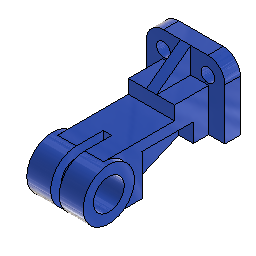
Design 12 v1 (Autodesk Fusion 360 design; units mm, degrees)
Autodesk Fusion 360 part; units mm, degrees
sketch "Sketch1" plane through (0, 0, 0) normal (1, 0, 0) x (0, 1, 0)
  circle A0 centre (0, 0) radius 180
  circle A1 centre (0, 0) radius 300
  line L0 (0, 300) -> (830, 300)
  line L1 (830, 300) -> (830, 460)
  line L2 (830, 460) -> (1230, 460)
  line L3 (1230, 460) -> (1230, -40)
  line L4 (1230, -40) -> (1050, -40)
  line L5 (1050, 180) -> (450, 180)
  line L6 (450, 180) -> (450, -300)
  line L7 (450, -300) -> (0, -300)
  line L8 (1050, 180) -> (1050, -40)
  line L9 (1230, -40) -> (1410, -40)
  line L10 (1410, -40) -> (1410, 760)
  line L11 (1410, 760) -> (1230, 760)
  line L12 (1230, 760) -> (1230, -40)
  line L13 (1230, 760) -> (830, 460)
  line L14 (450, -300) -> (1050, -40)
  dimension "d1" = 360
  dimension "d2" = 600
  dimension "d3" = 800
  dimension "d4" = 180
  dimension "d5" = 180
  dimension "d6" = 450
  dimension "d7" = 600
  dimension "d8" = 160
  dimension "d9" = 120
  dimension "d10" = 220
  dimension "d11" = 400
  dimension "d12" = 480
  constraint coincident A0.centre A1.centre
  constraint concentric A0 A1
  constraint coincident A1 L0.start
  constraint tangent A1 L0
  constraint horizontal L0
  constraint perpendicular L0 L1
  constraint perpendicular L1 L2
  constraint perpendicular L0 L3
  constraint perpendicular L1 L4
  constraint perpendicular L1 L5
  constraint perpendicular L5 L6
  constraint coincident A1 L7.end
  constraint tangent A1 L7
  constraint perpendicular L4 L8
  constraint horizontal L9
  constraint vertical L10
  constraint horizontal L11
  constraint vertical L12
  measures "d1" diameter of A0
  measures "d2" diameter of A1
  measures "d3" distance of L9.end L10.end
  measures "d4" distance of L3.end L9.end
  measures "d5" distance of L3.end L4.end
  measures "d6" horizontal distance of L6.end L7.end
  measures "d7" distance of L5.start L5.end
  measures "d8" distance of L0.end L1.end
  measures "d9" distance of L0 L5
  measures "d10" distance of L4.end L5.start
  measures "d11" distance of L1.end L2.end
  measures "d12" distance of L5.end L6.end
extrude "Extrude1" add sketch "Sketch1" along normal mid plane 660 contours A1
extrude "Extrude2" add sketch "Sketch1" along normal mid plane 540 contours A1 L0 L1 L2 L3 L4 L5 L6 L7 L8 L12
extrude "Extrude3" add sketch "Sketch1" along normal mid plane 120 contours L2 L12 L13
extrude "Extrude4" add sketch "Sketch1" along normal mid plane 920 contours L3 L9 L10 L11 L12
extrude "Extrude5" add sketch "Sketch1" along normal mid plane 200 contours L5 L6 L8 L14
fillet "Fillet1" radius 200 2 edges at (460, 1320, 760) (-460, 1320, 760)
sketch "Sketch2" plane through (0, 0, 300) normal (0, 0, 1) x (-1, 0, 0)
  line L0 (270, 0) -> (-270, 0)
  line L1 (-270, 0) -> (-270, -830)
  line L2 (-270, -830) -> (270, -830)
  line L3 (270, -830) -> (270, 0)
  line L4 (50, 314.5637) -> (-50, 314.5637)
  line L5 (-50, 314.5637) -> (-50, -314.5637)
  line L6 (-50, -314.5637) -> (50, -314.5637)
  line L7 (50, -314.5637) -> (50, 314.5637)
  line L8 (50, 314.5637) -> (-50, -314.5637) construction
  line L9 (-50, 314.5637) -> (50, -314.5637) construction
  point P0 (330, 300)
  point P1 (-330, 300)
  dimension "d25" = 100
  dimension "d26" = 280
  dimension "d27" = 280
  constraint horizontal L4
  constraint perpendicular L4 L5
  constraint parallel L4 L6
  constraint parallel L5 L7
  constraint coincident L8 origin
  constraint coincident L9 origin
  measures "d25" distance of L5.end L6.end
  measures "d26" distance of L7 P0
  measures "d27" horizontal distance of L4.end P1
extrude "Extrude6" cut sketch "Sketch2" against normal blind 1200 contours L0 L5 L6 L7 | L0 L4 L5 L7
hole "Hole1" at (260, 1230, 560) direction (0, 1, 0) diameter 160 end through all
mirror "Mirror1" about plane through (0, 0, 0) normal (1, 0, 0) of "Hole1"
